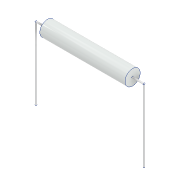
# Autodesk Inventor part: Reed Switch Puerta Derecha
Saved by Autodesk Inventor 2020 (Build 240168000, 168)
## iProperties
Created: 2020-08-13
Part Number: Reed Switch Puerta Derecha
Material: Aluminum 6061
Document SubType Name: Modeling
Designer: Dante
Density: 2.7 g/cm^3
Appearance: Aluminum - Flat
Author: Dante
Autodesk Inventor part; units mm, degrees
ref_plane "YZ Plane" through (0, 0, 0) normal (1, 0, 0) x (0, 1, 0)
ref_plane "XZ Plane" through (0, 0, 0) normal (0, 1, 0) x (-1, 0, 0)
ref_plane "XY Plane" through (0, 0, 0) normal (0, 0, 1) x (1, 0, 0)
sketch "Sketch2" plane through (0, 0, 0) normal (1, 0, 0) x (0, 1, 0)
  circle A0 centre (0, 0) radius 1.25
  dimension "d8" = 2.5
  constraints: 1 centre point
  measures "d8" diameter of A0
extrude "Extrusion1" add sketch "Sketch2" along normal blind 14
sketch "Sketch6" plane through (0, 0, 0) normal (0, 0, 1) x (1, 0, 0)
  line L0 (14, -1.25) -> (14, 1.25) projected
  line L1 (14, 0) -> (14, 0.125)
  line L2 (14, 0.125) -> (15.875, 0.125)
  line L3 (16, 0) -> (16, -11.875)
  line L4 (14, 0) -> (15.875, 0)
  line L5 (15.875, 0) -> (15.875, -11.875)
  line L6 (15.875, -11.875) -> (16, -11.875)
  line L7 (15.875, 0) -> (16, 0)
  line L8 (17.9417, 0) -> (15.75, 0)
  arc A0 (15.875, -0.125) -> (15.75, 0) centre (15.75, -0.125) ccw
  line L9 (15.75, 0) -> (16, 0)
  line L10 (0, 0) -> (0, 0.125)
  line L11 (0, 0.125) -> (-1.875, 0.125)
  line L12 (-2, 0) -> (-2, -11.875)
  line L13 (-2, -11.875) -> (-1.875, -11.875)
  line L14 (-1.875, -11.875) -> (-1.875, -0.125)
  line L15 (-1.75, 0) -> (0, 0)
  arc A1 (-1.875, 0.125) -> (-2, 0) centre (-1.875, 0) ccw
  arc A2 (-1.75, 0) -> (-1.875, -0.125) centre (-1.75, -0.125) ccw
  line L16 (-1.75, 0) -> (-2, 0)
  line L17 (-1.875, -0.125) -> (-1.875, 0)
  arc A3 (16, 0) -> (15.875, 0.125) centre (15.875, 0) ccw
  point P0 (16, 0.125)
  point P1 (18.875, 0.125)
  point P2 (-2, 0.125)
  point P3 (-1.875, 0)
  dimension "d16" = 0.125
  dimension "d17" = 2
  dimension "d18" = 12
  dimension "d19" = 1.875
  dimension "d26" = 0.125
  dimension "d27" = 2
  dimension "d28" = 0.125
  dimension "d29" = 0.125
  dimension "d30" = 0.125
  dimension "d33" = 0.125
  dimension "d35" = 12
  constraints: 34 end point, 9 point on circle, 9 point on line, 8 perpendicular, 7 tangent, 4 centre point, 4 vertical, 1 collinear, 1 horizontal, 1 midpoint
  measures "d16" distance of L1.start L1.end
  measures "d17" distance of L1.end point (16, 0.125)
  measures "d18" distance of point (16, 0.125) L3.end
  measures "d19" distance of L1.start L4.end
  measures "d26" distance of L10.start L10.end
  measures "d27" distance of L10.end point (-2, 0.125)
  measures "d28" distance of L12.end L13.end
  measures "d29" radius of A1
  measures "d30" radius of A2
  measures "d33" radius of A3
  measures "d35" distance between parallel lines of L13 L11
revolve "Revolution2" add sketch "Sketch6" angle 360 about axis through (14, 0, 0) along (1, 0, 0) contours L0 L2 A3 L7 L4
revolve "Revolution3" add sketch "Sketch6" angle 360 about axis through (15.875, 0, 0) along (0, -1, 0) contours L7 L3 L6 L5
revolve "Revolution4" add sketch "Sketch6" angle 360 about axis through (-1.75, 0, 0) along (1, 0, 0) contours L15 L16 A1 L11 L10
revolve "Revolution5" add sketch "Sketch6" angle 360 about axis through (-1.875, -11.875, 0) along (0, 1, 0) contours L14 L13 L12 L16 L17
equation "\"d27\" = d17"
equation "\"d35\" = d18"
body "Solid1"
